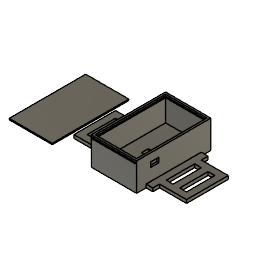
Sergio_TB_CaseV1 (Autodesk Fusion 360 design; units mm, degrees)
part number: 2026-03-08-13-35-21-563
Autodesk Fusion 360 part; units mm, degrees
sketch "Sketch1" plane through (0, 0, 0) normal (0, 0, 1) x (1, 0, 0)
  line L0 (-10, 20) -> (57.2, 20)
  line L1 (57.2, 20) -> (57.2, -90.2)
  line L2 (57.2, -90.2) -> (-10, -90.2)
  line L3 (-10, -90.2) -> (-10, 20)
  dimension "d1" = 67.2
  dimension "d2" = 110.2
  constraint horizontal L0
  constraint vertical L1
  constraint horizontal L2
  constraint vertical L3
  measures "d1" distance of L0.start L0.end
  measures "d2" distance of L0.start L2.end
extrude "Extrude1" add sketch "Sketch1" along normal blind 41.75 makes body 1
sketch "Sketch2" plane through (0, 0, 41.75) normal (0, 0, 1) x (-1, 0, 0)
  line L0 (10, 90.2) -> (-57.2, 90.2)
  line L1 (-57.2, 90.2) -> (-57.2, -20)
  line L2 (-57.2, -20) -> (10, -20)
  line L3 (10, -20) -> (10, 90.2)
  line L4 (7, -17) -> (-54.2, -17)
  line L5 (-54.2, -17) -> (-54.2, 87.2)
  line L6 (-54.2, 87.2) -> (7, 87.2)
  line L7 (7, 87.2) -> (7, -17)
  dimension "d10" = 61.2
  dimension "d11" = 104.2
  dimension "d12" = 3
  dimension "d13" = 3
  constraint horizontal L4
  constraint vertical L5
  constraint horizontal L6
  constraint vertical L7
  measures "d10" distance of L4.start L4.end
  measures "d11" distance of L4.end L5.end
  measures "d12" distance of L3 L7
  measures "d13" distance of L2 L4
extrude "Extrude3" cut sketch "Sketch2" against normal blind 36.75 contours L4 L5 L6 L7 bodies 1
sketch "Sketch4" plane through (0, -90.2, 0) normal (0, -1, 0) x (1, 0, 0)
  line L0 (-10, 0) -> (57.2, 0)
  line L1 (57.2, 0) -> (57.2, 41.75)
  line L2 (57.2, 41.75) -> (-10, 41.75)
  line L3 (-10, 41.75) -> (-10, 0)
  line L4 (-8.5, 39.25) -> (55.7, 39.25)
  line L5 (55.7, 39.25) -> (55.7, 37.25)
  line L6 (55.7, 37.25) -> (-8.5, 37.25)
  line L7 (-8.5, 37.25) -> (-8.5, 39.25)
  line L8 (54.2, 41.75) -> (-7, 41.75)
  line L9 (-131.921, 1.9) -> (-67.821, 1.9)
  line L10 (-67.821, 1.9) -> (-67.821, 0)
  line L11 (-67.821, 0) -> (-131.921, 0)
  line L12 (-131.921, 0) -> (-131.921, 1.9)
  dimension "d22" = 64.2
  dimension "d23" = 2
  dimension "d24" = 2.5
  dimension "d25" = 1.5
  dimension "d40" = 1.9
  dimension "d41" = 64.1
  constraint horizontal L4
  constraint vertical L5
  constraint horizontal L6
  constraint vertical L7
  constraint horizontal L9
  constraint vertical L10
  constraint horizontal L11
  constraint vertical L12
  constraint collinear L0 L11
  measures "d22" distance of L4.start L4.end
  measures "d23" distance of L4.start L6.end
  measures "d24" distance of L4 L8
  measures "d25" distance of L3 L7
  measures "d40" distance of L9 L11
  measures "d41" distance of L9.start L9.end
extrude "Extrude4" cut sketch "Sketch4" against normal blind 108.7 contours L4 L5 L6 L7 bodies 1
extrude "Extrude6" add sketch "Sketch4" against normal blind 113.7 separate body contours L9 L10 L11 L12 makes body 2
sketch "Sketch5" plane through (0, 0, 0) normal (0, 0, -1) x (1, 0, 0)
  line L0 (57.2, 90.2) -> (-10, 90.2)
  line L1 (-10, 90.2) -> (-10, -20)
  line L2 (-10, -20) -> (57.2, -20)
  line L3 (-10, 4.1) -> (-60, 4.1)
  line L4 (-60, 4.1) -> (-60, 66.1)
  line L5 (-60, 66.1) -> (-10, 66.1)
  line L6 (-10, 66.1) -> (-10, 4.1)
  line L7 (57.2, -20) -> (-10, -20)
  line L8 (-50, 14.1) -> (-40, 14.1)
  line L9 (-40, 14.1) -> (-40, 56.1)
  line L10 (-40, 56.1) -> (-50, 56.1)
  line L11 (-50, 56.1) -> (-50, 14.1)
  line L12 (-30, 14.1) -> (-20, 14.1)
  line L13 (-20, 14.1) -> (-20, 56.1)
  line L14 (-20, 56.1) -> (-30, 56.1)
  line L15 (-30, 56.1) -> (-30, 14.1)
  line L16 (23.6, -15.6534) -> (23.6, 85)
  line L17 (-10, -20) -> (-10, 90.2)
  line L18 (87.2, 14.1) -> (87.2, 56.1)
  line L19 (77.2, 56.1) -> (77.2, 14.1)
  line L20 (77.2, 14.1) -> (67.2, 14.1)
  line L21 (57.2, 4.1) -> (107.2, 4.1)
  line L22 (87.2, 56.1) -> (97.2, 56.1)
  line L23 (67.2, 14.1) -> (67.2, 56.1)
  line L24 (57.2, 66.1) -> (57.2, 4.1)
  line L25 (67.2, 56.1) -> (77.2, 56.1)
  line L26 (107.2, 4.1) -> (107.2, 66.1)
  line L27 (97.2, 56.1) -> (97.2, 14.1)
  line L28 (107.2, 66.1) -> (57.2, 66.1)
  line L29 (97.2, 14.1) -> (87.2, 14.1)
  line L30 (-10, 4.1) -> (-20, 4.1)
  line L31 (-20, 4.1) -> (-20, -5.9)
  line L32 (-20, -5.9) -> (-10, -5.9)
  line L33 (-10, -5.9) -> (-10, 4.1)
  line L34 (-10, 66.1) -> (-20, 66.1)
  line L35 (-20, 66.1) -> (-20, 76.1)
  line L36 (-20, 76.1) -> (-10, 76.1)
  line L37 (-10, 76.1) -> (-10, 66.1)
  line L38 (87.2, 56.1) -> (97.2, 56.1)
  line L39 (67.2, 76.1) -> (57.2, 76.1)
  line L40 (57.2, 66.1) -> (67.2, 66.1)
  line L41 (87.2, 14.1) -> (87.2, 56.1)
  line L42 (57.2, 4.1) -> (107.2, 4.1)
  line L43 (67.2, -5.9) -> (57.2, -5.9)
  line L44 (97.2, 14.1) -> (87.2, 14.1)
  line L45 (77.2, 56.1) -> (77.2, 14.1)
  line L46 (67.2, 66.1) -> (67.2, 76.1)
  line L47 (57.2, 4.1) -> (67.2, 4.1)
  line L48 (77.2, 14.1) -> (67.2, 14.1)
  line L49 (107.2, 66.1) -> (57.2, 66.1)
  line L50 (57.2, 66.1) -> (57.2, 4.1)
  line L51 (57.2, -5.9) -> (57.2, 4.1)
  line L52 (67.2, 56.1) -> (77.2, 56.1)
  line L53 (67.2, 14.1) -> (67.2, 56.1)
  line L54 (97.2, 56.1) -> (97.2, 14.1)
  line L55 (57.2, 76.1) -> (57.2, 66.1)
  line L56 (67.2, 4.1) -> (67.2, -5.9)
  dimension "d28" = 24.1
  dimension "d29" = 62
  dimension "d30" = 50
  dimension "d31" = 42
  dimension "d32" = 10
  dimension "d34" = 10
  dimension "d35" = 10
  dimension "d36" = 10
  dimension "d37" = 33.6
  dimension "d44" = 10
  dimension "d45" = 10
  dimension "d46" = 10
  dimension "d47" = 10
  constraint horizontal L3
  constraint vertical L4
  constraint horizontal L5
  constraint vertical L6
  constraint coincident L1 L3.start
  constraint horizontal L8
  constraint vertical L9
  constraint horizontal L10
  constraint vertical L11
  constraint horizontal L12
  constraint vertical L13
  constraint horizontal L14
  constraint vertical L15
  constraint equal L8 L12
  constraint equal L11 L15
  constraint collinear L8 L12
  constraint perpendicular L7 L16
  constraint symmetric L3.start L16 L21.start
  constraint symmetric L3.end L16 L21.end
  constraint symmetric L4.end L16 L26.end
  constraint symmetric L5.end L16 L24.start
  constraint symmetric L8.start L16 L27.end
  constraint symmetric L8.end L16 L18.start
  constraint symmetric L9.end L16 L18.end
  constraint symmetric L10.end L16 L22.end
  constraint symmetric L12.start L16 L19.end
  constraint symmetric L12.end L16 L20.end
  constraint symmetric L13.end L16 L23.end
  constraint symmetric L14.end L16 L19.start
  constraint horizontal L30
  constraint vertical L31
  constraint horizontal L32
  constraint vertical L33
  constraint horizontal L34
  constraint vertical L35
  constraint horizontal L36
  constraint vertical L37
  constraint symmetric L16 L30.end L47.end
  constraint symmetric L16 L31.end L43.start
  constraint symmetric L16 L32.end L43.end
  constraint symmetric L16 L34.end L40.end
  constraint symmetric L16 L35.end L39.start
  constraint symmetric L16 L36.end L39.end
  measures "d28" distance of L3 L7
  measures "d29" distance of L3.end L4.end
  measures "d30" distance of L3.start L3.end
  measures "d31" distance of L8.start L10.end
  measures "d32" distance of L8.start L8.end
  measures "d34" distance of L9 L15
  measures "d35" distance of L4 L11
  measures "d36" distance of L3 L8
  measures "d37" distance of L16 L17
  measures "d44" distance of L3.start L30.end
  measures "d45" distance of L3.start L32.end
  measures "d46" distance of L5.end L34.end
  measures "d47" distance of L5.end L36.end
extrude "Extrude5" add sketch "Sketch5" against normal blind 5 bodies 1
sketch "Sketch7" plane through (0, 0, 5) normal (0, 0, 1) x (-1, 0, 0)
  line L0 (7, 87.2) -> (-54.2, 87.2)
  line L1 (-54.2, 87.2) -> (-54.2, -17)
  line L2 (-54.2, -17) -> (7, -17)
  line L3 (7, -17) -> (7, 87.2)
  line L4 (-13.5, 29) -> (-23.5, 29)
  line L5 (-23.5, 29) -> (-23.5, 39)
  line L6 (-23.5, 39) -> (-13.5, 39)
  line L7 (-13.5, 39) -> (-13.5, 29)
  dimension "d48" = 46
  dimension "d49" = 20.5
  dimension "d50" = 10
  dimension "d51" = 10
  constraint horizontal L4
  constraint vertical L5
  constraint horizontal L6
  constraint vertical L7
  measures "d48" distance of L2 L4
  measures "d49" distance of L3 L7
  measures "d50" distance of L4.start L4.end
  measures "d51" distance of L4.end L5.end
extrude "Extrude7" cut sketch "Sketch7" against normal blind 5 contours L4 L5 L6 L7 bodies 1
sketch "Sketch8" plane through (54.2, 0, 0) normal (-1, 0, 0) x (0, -1, 0)
  line L0 (87.2, 37.25) -> (-17, 37.25)
  line L1 (-17, 37.25) -> (-17, 5)
  line L2 (-17, 5) -> (87.2, 5)
  line L3 (87.2, 5) -> (87.2, 37.25)
  line L4 (57.15, 30.05) -> (69.25, 30.05)
  line L5 (69.25, 30.05) -> (69.25, 22.95)
  line L6 (69.25, 22.95) -> (57.15, 22.95)
  line L7 (57.15, 22.95) -> (57.15, 30.05)
  dimension "d54" = 17.95
  dimension "d55" = 17.95
  dimension "d56" = 12.1
  dimension "d57" = 7.1
  constraint horizontal L4
  constraint vertical L5
  constraint horizontal L6
  constraint vertical L7
  measures "d54" distance of L3 L5
  measures "d55" distance of L2 L6
  measures "d56" distance of L4.start L4.end
  measures "d57" distance of L4.end L5.end
extrude "Extrude8" cut sketch "Sketch8" against normal blind 3 contours L4 L5 L6 L7 bodies 1
equation "d40 = 2 mm - 0.1 mm"
equation "d41 = 64.2 mm - 0.1 mm"
equation "d54 = 1.8 cm - 0.05 mm"
equation "d55 = 18 mm - 0.05 mm"
equation "d56 = 1.2 cm + 0.1 mm"
equation "d57 = 7 mm + 0.1 mm"
